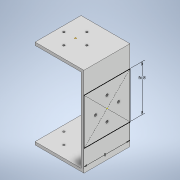
# Autodesk Inventor part: sidebracket
Saved by Autodesk Inventor 2022.2 (Build 262287030, 287C)
## iProperties
Created: 2022-03-11
Part Number: sidebracket
Material: Generic
Document SubType Name: Modeling
Designer: Tapendra
Density: 1 g/cm^3
Appearance: Default
Author: Tapendra
Autodesk Inventor part; units mm, degrees
ref_plane "YZ Plane" through (0, 0, 0) normal (1, 0, 0) x (0, 1, 0)
ref_plane "XZ Plane" through (0, 0, 0) normal (0, 1, 0) x (-1, 0, 0)
ref_plane "XY Plane" through (0, 0, 0) normal (0, 0, 1) x (1, 0, 0)
sketch "Sketch1" plane through (0, 0, 0) normal (0, 0, 1) x (1, 0, 0)
  line L0 (20.183, 72.5) -> (20.183, -72.5)
  line L1 (20.183, 72.5) -> (165.183, 72.5) construction
  line L2 (20.183, -72.5) -> (-59.817, -72.5)
  line L3 (-59.817, -72.5) -> (-59.817, -77.5)
  line L4 (-59.817, -72.5) -> (-54.817, -72.5) construction
  line L5 (-59.817, -77.5) -> (25.183, -77.5)
  line L6 (25.183, -77.5) -> (25.183, 77.5)
  line L7 (25.183, 77.5) -> (-59.817, 77.5)
  line L8 (-59.817, 77.5) -> (-59.817, 72.5)
  line L9 (-59.817, 72.5) -> (20.183, 72.5)
  point P0 (0, 0)
  dimension "d0" = 145
  dimension "d1" = 90
  dimension "d2" = 80
  dimension "d3" = 90
  dimension "d4" = 5
  dimension "d5" = 90
  dimension "d6" = 85
  dimension "d7" = 90
  dimension "d8" = 155
  dimension "d9" = 90
  dimension "d10" = 85
  dimension "d11" = 90
  dimension "d12" = 5
  dimension "d13" = 90
  dimension "d45" = 72.5
  constraints: 20 end point, 7 perpendicular, 2 horizontal, 2 vertical
  measures "d0" distance of L0.start L0.end
  measures "d1" angle of L0 L1
  measures "d2" distance of L0.end L2.end
  measures "d3" angle of L0 L2
  measures "d4" distance of L2.end L3.end
  measures "d5" angle of L3 L4
  measures "d6" distance of L3.end L5.end
  measures "d7" angle of L5 L3
  measures "d8" distance of L5.end L6.end
  measures "d9" angle of L6 L5
  measures "d10" distance of L6.end L7.end
  measures "d11" angle of L7 L6
  measures "d12" distance of L7.end L8.end
  measures "d13" angle of L8 L7
  measures "d45" distance from line of L2 point (0, 0)
extrude "Extrusion1" add sketch "Sketch1" along normal mid plane 80
sketch "Sketch2" plane through (25.183, -77.5, 40) normal (1, 0, 0) x (0, 0, -1)
  line L0 (0, 0) -> (0, 155) projected
  line L1 (0, 150) -> (0, 5) projected
  line L2 (0, 77.5) -> (80, 77.5) construction
  line L3 (80, 5) -> (80, 150) projected
  line L4 (80, 0) -> (0, 0) projected
  line L5 (40, 37.5) -> (40, 117.5) construction
  line L6 (80, 77.5) -> (0, 77.5) construction
  line L7 (40, 117.5) -> (40, 37.5) construction
  point P0 (40, 77.5)
  point P1 (40, 97.5)
  point P2 (40, 77.5)
  point P3 (40, 77.5)
  point P4 (20, 77.5)
  point P5 (40, 77.5)
  point P6 (40, 57.5)
  point P7 (40, 77.5)
  point P8 (60, 77.5)
  dimension "d16" = 40
  dimension "d17" = 77.5
  dimension "d18" = 20
  dimension "d21" = 360
  constraints: 8 end point, 3 midpoint, 2 coincident, 1 horizontal, 19 other
  measures "d16" distance from line of L0 point (40, 97.5)
  measures "d17" distance between parallel lines of L4 L2
  measures "d18" distance of point (40, 97.5) point (40, 77.5)
hole "Hole1" at (25.183, 20, 0) at (25.183, 0, 20) at (25.183, -20, 0) at (25.183, 0, -20) direction (-1, 0, 0) diameter 4.134 end through all thread size "M5x0.8" class "6H" standard "ANSI Metric M Profile"
sketch "Sketch3" plane through (-59.817, 77.5, 40) normal (0, 1, 0) x (1, 0, 0)
  line L0 (60, 80) -> (0, 80)
  line L1 (30, 80) -> (30, 0) construction
  line L2 (60, 0) -> (0, 0)
  line L3 (30, 80) -> (120, 80) construction
  line L4 (85, 80) -> (85, 0) projected
  line L5 (85, 0) -> (0, 0) projected
  line L6 (0, 80) -> (85, 80) projected
  point P0 (59.817, 40)
  point P1 (10, 40)
  point P2 (30, 40)
  point P3 (30, 20)
  point P4 (50, 40)
  point P5 (30, 60)
  dimension "d30" = 90
  dimension "d31" = 55
  dimension "d32" = 40
  dimension "d33" = 20
  dimension "d36" = 360
  constraints: 8 end point, 3 midpoint, 2 point on line, 1 horizontal, 5 other
  measures "d30" angle of L1 L3
  measures "d31" distance between parallel lines of L4 L1
  measures "d32" distance from line of L2 point (10, 40)
  measures "d33" distance from line of point (10, 40) L1
hole "Hole2" at (-9.817, 77.5, 0) at (-29.817, 77.5, 20) at (-49.817, 77.5, 0) at (-29.817, 77.5, -20) direction (0, -1, 0) diameter 3.302 end through all thread size "8-32 UNC" class "2B" standard "ANSI Unified Screw Threads"
sketch "Sketch4" plane through (25.183, -77.5, 40) normal (1, 0, 0) x (0, 0, -1)
  line L0 (0, 117.5) -> (80, 117.5)
  line L1 (80, 117.5) -> (80, 37.5)
  line L2 (80, 37.5) -> (0, 37.5)
  line L3 (0, 37.5) -> (0, 117.5)
  line L4 (0, 117.5) -> (80, 37.5) construction
  line L5 (80, 117.5) -> (0, 37.5) construction
  point P0 (40, 77.5)
  dimension "d46" = 80
  dimension "d47" = 80
  constraints: 12 end point, 2 midpoint, 2 parallel, 1 horizontal, 1 perpendicular
  measures "d46" distance of L1.end L2.end
  measures "d47" distance of L0.end L1.end
equation "\"d47\" = d46"
body "Solid1"
